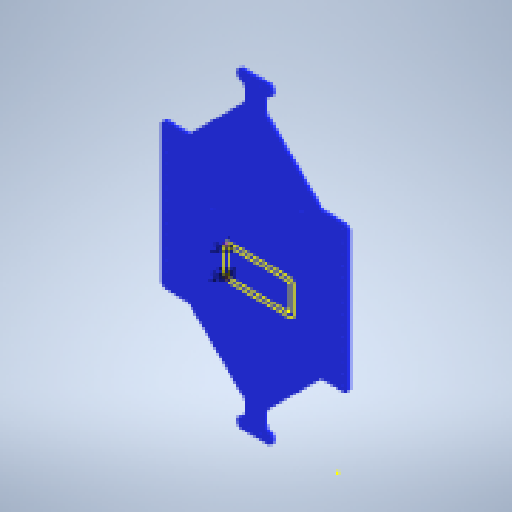
# Autodesk Inventor part: BPlate
Saved by Autodesk Inventor 2024 (Build 280153000, 153)
## iProperties
Created: 2024-01-06
Part Number: BPlate
Material: Polycarbonate, Clear
Document SubType Name: Modeling
Designer: student
Density: 1.2 g/cm^3
Appearance: Blue - Wall Paint - Glossy
Author: student
Autodesk Inventor part; units mm, degrees
ref_plane "YZ Plane" through (0, 0, 0) normal (1, 0, 0) x (0, 1, 0)
ref_plane "XZ Plane" through (0, 0, 0) normal (0, 1, 0) x (-1, 0, 0)
sketch "Sketch1" plane through (0, 0, 0) normal (0, 0, 1) x (1, 0, 0)
  circle A0 centre (-241.3, -12.7) radius 1.5875 projected
  circle A1 centre (-215.9, -12.7) radius 1.5875 projected
  circle A2 centre (-190.5, -12.7) radius 1.5875 projected
  circle A3 centre (-165.1, -12.7) radius 1.5875 projected
  circle A4 centre (12.7, 520.7) radius 1.5875 projected
  circle A5 centre (12.7, 495.3) radius 1.5875 projected
  circle A6 centre (12.7, 469.9) radius 1.5875 projected
  circle A7 centre (12.7, 444.5) radius 1.5875 projected
  circle A8 centre (12.7, 419.1) radius 1.5875 projected
  circle A9 centre (12.7, 393.7) radius 1.5875 projected
  circle A10 centre (12.7, 368.3) radius 1.5875 projected
  circle A11 centre (12.7, 342.9) radius 1.5875 projected
  circle A12 centre (12.7, 317.5) radius 1.5875 projected
  circle A13 centre (12.7, 292.1) radius 1.5875 projected
  circle A14 centre (12.7, 266.7) radius 1.5875 projected
  circle A15 centre (12.7, 241.3) radius 1.5875 projected
  circle A16 centre (12.7, 215.9) radius 1.5875 projected
  circle A17 centre (12.7, 190.5) radius 1.5875 projected
  circle A18 centre (-419.1, 190.5) radius 1.5875 projected
  circle A19 centre (-419.1, 215.9) radius 1.5875 projected
  circle A20 centre (-419.1, 241.3) radius 1.5875 projected
  circle A21 centre (-419.1, 266.7) radius 1.5875 projected
  circle A22 centre (-419.1, 292.1) radius 1.5875 projected
  circle A23 centre (-419.1, 317.5) radius 1.5875 projected
  circle A24 centre (-419.1, 342.9) radius 1.5875 projected
  circle A25 centre (-419.1, 368.3) radius 1.5875 projected
  circle A26 centre (-419.1, 393.7) radius 1.5875 projected
  circle A27 centre (-419.1, 419.1) radius 1.5875 projected
  circle A28 centre (-419.1, 444.5) radius 1.5875 projected
  circle A29 centre (-419.1, 469.9) radius 1.5875 projected
  circle A30 centre (-419.1, 495.3) radius 1.5875 projected
  circle A31 centre (-419.1, 520.7) radius 1.5875 projected
  circle A32 centre (-165.1, 723.9) radius 1.5875 projected
  circle A33 centre (-190.5, 723.9) radius 1.5875 projected
  circle A34 centre (-215.9, 723.9) radius 1.5875 projected
  circle A35 centre (-241.3, 723.9) radius 1.5875 projected
  line L0 (-165.1, 723.9) -> (-241.3, 723.9)
  line L1 (-165.1, -12.7) -> (-241.3, -12.7)
  line L2 (-419.1, 520.7) -> (-419.1, 190.5)
  line L3 (-406.4, 177.8) -> (-431.8, 177.8)
  line L4 (-431.8, 177.8) -> (-431.8, 533.4)
  line L5 (-431.8, 533.4) -> (-406.4, 533.4)
  line L6 (-406.4, 533.4) -> (-406.4, 177.8)
  line L7 (-406.4, 177.8) -> (-431.8, 533.4) construction
  line L8 (-431.8, 177.8) -> (-406.4, 533.4) construction
  circle A36 centre (12.7, 190.5) radius 1.5875
  circle A37 centre (12.7, 215.9) radius 1.5875
  circle A38 centre (12.7, 241.3) radius 1.5875
  circle A39 centre (12.7, 266.7) radius 1.5875
  circle A40 centre (12.7, 292.1) radius 1.5875
  circle A41 centre (12.7, 317.5) radius 1.5875
  circle A42 centre (12.7, 342.9) radius 1.5875
  circle A43 centre (12.7, 368.3) radius 1.5875
  circle A44 centre (12.7, 393.7) radius 1.5875
  circle A45 centre (12.7, 419.1) radius 1.5875
  circle A46 centre (12.7, 444.5) radius 1.5875
  circle A47 centre (12.7, 469.9) radius 1.5875
  circle A48 centre (12.7, 495.3) radius 1.5875
  circle A49 centre (12.7, 520.7) radius 1.5875
  line L9 (25.4, 177.8) -> (0, 177.8)
  line L10 (0, 533.4) -> (25.4, 533.4)
  line L11 (25.4, 533.4) -> (25.4, 177.8)
  line L12 (25.4, 177.8) -> (0, 533.4) construction
  line L13 (0, 177.8) -> (25.4, 533.4) construction
  line L14 (12.7, 190.5) -> (12.7, 520.7)
  line L15 (-247.65, 0) -> (-247.65, -25.4)
  line L16 (-247.65, -25.4) -> (-158.75, -25.4)
  line L17 (-158.75, -25.4) -> (-158.75, 0)
  line L18 (-158.75, 0) -> (-247.65, -25.4) construction
  line L19 (-247.65, 0) -> (-158.75, -25.4) construction
  line L20 (-247.65, 711.2) -> (-158.75, 711.2)
  line L21 (-158.75, 711.2) -> (-158.75, 736.6)
  line L22 (-158.75, 736.6) -> (-247.65, 736.6)
  line L23 (-247.65, 736.6) -> (-247.65, 711.2)
  line L24 (-247.65, 711.2) -> (-158.75, 736.6) construction
  line L25 (-158.75, 711.2) -> (-247.65, 736.6) construction
  line L26 (-228.6, 0) -> (-177.8, 0)
  line L27 (0, 492.125) -> (0, 533.4)
  line L28 (-41.275, 177.8) -> (-177.8, 41.275)
  line L29 (-177.8, 669.925) -> (-41.275, 533.4)
  line L30 (-228.6, 669.925) -> (-365.125, 533.4)
  line L31 (-365.125, 177.8) -> (-228.6, 41.275)
  line L32 (-177.8, 669.925) -> (-177.8, 711.2)
  line L33 (0, 533.4) -> (-41.275, 533.4)
  line L34 (-228.6, 711.2) -> (-228.6, 669.925)
  line L35 (-177.8, 533.4) -> (-228.6, 533.4)
  line L36 (-365.125, 533.4) -> (-406.4, 533.4)
  line L37 (-406.4, 177.8) -> (-365.125, 177.8)
  line L38 (-228.6, 533.4) -> (-228.6, 177.8)
  line L39 (-228.6, 41.275) -> (-228.6, 0)
  line L40 (-177.8, 0) -> (-177.8, 41.275)
  line L41 (-177.8, 177.8) -> (-177.8, 533.4)
  line L42 (-228.6, 177.8) -> (-177.8, 177.8)
  line L43 (-41.275, 177.8) -> (0, 177.8)
  line L44 (0, 177.8) -> (0, 219.075)
  line L45 (0, 492.125) -> (0, 533.4)
  line L46 (-158.75, 0) -> (-177.8, 0)
  line L47 (-228.6, 0) -> (-247.65, 0)
  line L48 (-177.8, 711.2) -> (-187.325, 711.2)
  line L49 (-219.075, 711.2) -> (-228.6, 711.2)
  line L50 (-406.4, 533.4) -> (-406.4, 492.125)
  line L51 (-406.4, 219.075) -> (-406.4, 177.8)
  point P0 (0, 0)
  point P1 (-419.1, 355.6)
  point P2 (12.7, 355.6)
  point P3 (-203.2, -12.7)
  point P4 (-203.2, 723.9)
  point P5 (-203.2, -25.4)
  dimension "d0" = 25.4
  dimension "d1" = 355.6
  dimension "d2" = 25.4
  dimension "d3" = 355.6
  dimension "d4" = 88.9
  dimension "d5" = 25.4
  dimension "d6" = 88.9
  dimension "d7" = 25.4
  dimension "d11" = 66.675
  dimension "d12" = 66.675
  dimension "d13" = 66.675
  dimension "d14" = 66.675
  dimension "d15" = 66.675
  dimension "d16" = 66.675
  dimension "d17" = 66.675
  dimension "d18" = 66.675
  constraints: 104 end point, 32 parallel, 14 centre point, 13 perpendicular, 12 midpoint, 11 horizontal, 7 point on line, 2 collinear, 1 vertical, 1 other
  measures "d0" distance of L4.end L5.end
  measures "d1" distance between parallel lines of L3 L5
  measures "d2" distance of L10.start L10.end
  measures "d3" distance between parallel lines of L9 L10
  measures "d4" distance of L16.end L15.end
  measures "d5" distance of L15.end L15.start
  measures "d6" distance of L22.end L21.end
  measures "d7" distance of L21.end L20.end
  measures "d11" distance of L11.end L28.start
  measures "d12" distance from line of L16 L28.end
  measures "d13" distance from line of L11 L29.end
  measures "d14" distance from line of L22 L29.start
  measures "d15" distance from line of L16 L31.end
  measures "d16" distance of L3.end L31.start
  measures "d17" distance from line of L4 L30.end
  measures "d18" distance from line of L22 L30.start
extrude "Extrusion1" add sketch "Sketch1" along normal blind 6.35 contours L3 L4 L5 L6 | L6 L36 L30 L34 L20 L32 L29 L33 L10 L11 L9 L43 L28 L40 L26 L39 L31 L37 | L26 L46 L17 L16 L15 L47 | L20 L23 L22 L21 | L41 L42 L38 L35
fillet "Fillet1" radius 12.7 24 edges at (-228.6, 41.275, 3.175) (-228.6, 0, 3.175) (-247.65, 0, 3.175) (-247.65, -25.4, 3.175) (-158.75, -25.4, 3.175) (-177.8, 0, 3.175) (-158.75, 0, 3.175) (-177.8, 41.275, 3.175) (-41.275, 177.8, 3.175) (25.4, 177.8, 3.175) (25.4, 533.4, 3.175) (-41.275, 533.4, 3.175) (-177.8, 669.925, 3.175) (-177.8, 711.2, 3.175) (-158.75, 711.2, 3.175) (-158.75, 736.6, 3.175) (-247.65, 736.6, 3.175) (-247.65, 711.2, 3.175) (-228.6, 711.2, 3.175) (-228.6, 669.925, 3.175) (-365.125, 533.4, 3.175) (-365.125, 177.8, 3.175) (-431.8, 177.8, 3.175) (-431.8, 533.4, 3.175)
sketch "Sketch2" plane through (0, 0, 0) normal (0, 0, -1) x (-1, 0, 0)
  circle A0 centre (304.7995, 406.4002) radius 2.5 projected
  circle A1 centre (89.1163, 508.4596) radius 2.5 projected
  point P0 (0, 0)
extrude "Extrusion2" cut sketch "Sketch2" against normal blind 6.35
ref_plane "Work Plane1" through (-203.2, 190.5, 0) normal (1, 0, 0) x (0, 0, -1)
sketch "Sketch3" plane through (0, 0, 6.35) normal (0, 0, 1) x (1, 0, 0)
  arc A0 (-279.4, 282.44) -> (-267.74, 270.78) centre (-267.74, 282.44) ccw projected
  line L0 (-279.4, 343.94) -> (-279.4, 282.44) projected
  arc A1 (-267.74, 355.6) -> (-279.4, 343.94) centre (-267.74, 343.94) ccw projected
  line L1 (-119.74, 355.6) -> (-267.74, 355.6) projected
  arc A2 (-108.08, 343.94) -> (-119.74, 355.6) centre (-119.74, 343.94) ccw projected
  line L2 (-108.08, 282.44) -> (-108.08, 343.94) projected
  arc A3 (-119.74, 270.78) -> (-108.08, 282.44) centre (-119.74, 282.44) ccw projected
  line L3 (-267.74, 270.78) -> (-119.74, 270.78) projected
  line L4 (-119.74, 280.94) -> (-267.74, 280.94) projected
  arc A4 (-119.74, 280.94) -> (-118.24, 282.44) centre (-119.74, 282.44) ccw projected
  line L5 (-118.24, 343.94) -> (-118.24, 282.44) projected
  arc A5 (-118.24, 343.94) -> (-119.74, 345.44) centre (-119.74, 343.94) ccw projected
  line L6 (-267.74, 345.44) -> (-119.74, 345.44) projected
  arc A6 (-267.74, 345.44) -> (-269.24, 343.94) centre (-267.74, 343.94) ccw projected
  line L7 (-269.24, 282.44) -> (-269.24, 343.94) projected
  arc A7 (-269.24, 282.44) -> (-267.74, 280.94) centre (-267.74, 282.44) ccw projected
  circle A8 centre (-271.78, 278.4) radius 2.54
  circle A9 centre (-271.78, 347.98) radius 2.54
  circle A10 centre (-115.7, 278.4) radius 2.54
  circle A11 centre (-115.7, 347.98) radius 2.54
  point P0 (0, 0)
  dimension "d24" = 5.08
  dimension "d26" = 5.08
  dimension "d27" = 5.08
  dimension "d28" = 5.08
  dimension "d29" = 7.62
  dimension "d30" = 7.62
  dimension "d31" = 7.62
  dimension "d32" = 7.62
  dimension "d33" = 7.62
  dimension "d34" = 7.62
  dimension "d35" = 7.62
  dimension "d36" = 7.62
  constraints: 4 centre point, 1 tangent
  measures "d24" diameter of A8
  measures "d26" diameter of A9
  measures "d27" diameter of A10
  measures "d28" diameter of A11
  measures "d29" distance from line of L3 A10.centre
  measures "d30" distance from line of L2 A10.centre
  measures "d31" distance from line of L2 A11.centre
  measures "d32" distance from line of L1 A11.centre
  measures "d33" distance from line of L1 A9.centre
  measures "d34" distance from line of L0 A9.centre
  measures "d35" distance from line of L0 A8.centre
  measures "d36" distance from line of L3 A8.centre
extrude "Extrusion3" cut sketch "Sketch3" against normal through all contours A8 | A9 | A10 | A11
equation "\"d12\" = d11"
equation "\"d13\" = d11"
equation "\"d14\" = d11"
equation "\"d15\" = d12"
equation "\"d16\" = d15"
equation "\"d17\" = d11"
equation "\"d18\" = d11"
body "Solid1"
